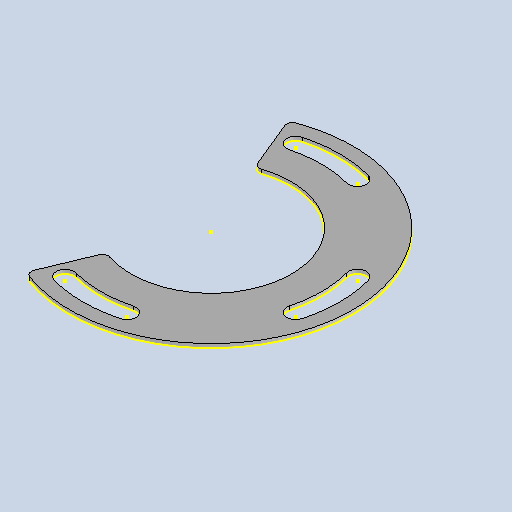
# Autodesk Inventor part: PNS 1707 funnel flange
Saved by Autodesk Inventor 2025.3 (Build 293356030, 356C)
## iProperties
Created: 2025-02-13
Part Number: PNS 1707 funnel flange
Material: Steel
Document SubType Name: Sheet Metal
Designer: admin
Mass: 720.962 g
Surface Area: 520.66 cm^2
Volume: 91.8424 cm^3
Density: 7.85 g/cm^3
Flat Pattern Width: 24.0684 cm
Flat Pattern Length: 28.4868 cm
Flat Pattern Area: 685.632 cm^2
Sheet Metal Rule: AISI304 4mm Die 32
Sheet Metal Width: 240,684 mm
Sheet Metal Length: 284,868 mm
Sheet Metal Area: 68563,227 mm^2
Appearance: Default
Author: pokla
Autodesk Inventor part; units mm, degrees
ref_plane "YZ Plane" through (0, 0, 0) normal (1, 0, 0) x (0, 1, 0)
ref_plane "XZ Plane" through (0, 0, 0) normal (0, 1, 0) x (-1, 0, 0)
ref_plane "XY Plane" through (0, 0, 0) normal (0, 0, 1) x (1, 0, 0)
sketch "Sketch2" plane through (0, 0, 0) normal (0, 0, 1) x (1, 0, 0)
  circle A0 centre (0, 0) radius 80.5
  circle A1 centre (0, 0) radius 142.5
  line L0 (0, 0) -> (-54.5324, 131.6528)
  line L1 (0, 0) -> (-54.5324, -131.6528)
  line L2 (0, 0) -> (-142.5, 0) construction
  point P0 (-30.806, -74.3723)
  point P1 (-30.806, 74.3723)
  dimension "d25" = 161
  dimension "d27" = 285
  dimension "d29" = 135
  measures "d25" diameter of A0
  measures "d27" diameter of A1
  measures "d29" angle of L1 L0
extrude "Plate2" add sketch "Sketch2" along normal blind 4 contours A0 L0 A1 L1 picked at (65.8732, 102.2302)
sketch "Sketch3" plane through (0, 0, 4) normal (0, 0, 1) x (1, 0, 0)
  circle A0 centre (0, 0) radius 120 construction
  arc A1 (31.0583, 115.9111) -> (-31.0583, 115.9111) centre (0, 0) ccw construction
  arc A2 (33.3877, 124.6044) -> (-33.3877, 124.6044) centre (0, 0) ccw
  arc A3 (28.7289, 107.2178) -> (-28.7289, 107.2178) centre (0, 0) ccw
  arc A4 (28.7289, 107.2178) -> (33.3877, 124.6044) centre (31.0583, 115.9111) ccw
  arc A5 (-33.3877, 124.6044) -> (-28.7289, 107.2178) centre (-31.0583, 115.9111) ccw
  line L0 (-31.0583, 115.9111) -> (0, 0)
  line L1 (0, 0) -> (31.0583, 115.9111)
  line L2 (0, 0) -> (0, 70.9879)
  dimension "d28" = 240
  dimension "d30" = 18
  dimension "d31" = 30
  constraints: 10 point on circle, 6 end point, 5 centre point, 4 tangent, 2 coincident, 1 vertical, 5 other
  measures "d30" diameter of A4
  measures "d31" angle of L1 L0
extrude "Cut1" cut sketch "Sketch3" against normal blind 4 contours A4 A3 A5 A2
pattern_circular "Circular Pattern1" count 4 over 360 about axis through (0, 0, 0) along (0, 0, 1) of "Cut1"
fillet "Corner Round1" radius 6 4 edges at (-54.5324, 131.6528, 2) (-30.806, 74.3723, 2) (-30.806, -74.3723, 2) (-54.5324, -131.6528, 2)
sketch "Sketch5" plane through (0, 0, 0) normal (0, 0, -1) x (-1, 0, 0)
  arc A0 (-107.2178, 28.7289) -> (-107.2178, -28.7289) centre (0, 0) ccw projected
  arc A1 (-124.6044, -33.3877) -> (-107.2178, -28.7289) centre (-115.9111, -31.0583) ccw projected
  arc A2 (-124.6044, 33.3877) -> (-124.6044, -33.3877) centre (0, 0) ccw projected
  arc A3 (-107.2178, 28.7289) -> (-124.6044, 33.3877) centre (-115.9111, 31.0583) ccw projected
  arc A4 (-28.7289, -107.2178) -> (28.7289, -107.2178) centre (0, 0) ccw projected
  arc A5 (33.3877, -124.6044) -> (28.7289, -107.2178) centre (31.0583, -115.9111) ccw projected
  arc A6 (-33.3877, -124.6044) -> (33.3877, -124.6044) centre (0, 0) ccw projected
  arc A7 (-28.7289, -107.2178) -> (-33.3877, -124.6044) centre (-31.0583, -115.9111) ccw projected
  arc A8 (28.7289, 107.2178) -> (-28.7289, 107.2178) centre (0, 0) ccw projected
  arc A9 (-33.3877, 124.6044) -> (-28.7289, 107.2178) centre (-31.0583, 115.9111) ccw projected
  arc A10 (33.3877, 124.6044) -> (-33.3877, 124.6044) centre (0, 0) ccw projected
  arc A11 (28.7289, 107.2178) -> (33.3877, 124.6044) centre (31.0583, 115.9111) ccw projected
  arc A12 (48.6927, -133.9226) -> (52.1858, -125.9877) centre (46.6425, -128.2838) ccw projected
  line L0 (33.0224, -79.7231) -> (52.1858, -125.9877) projected
  arc A13 (33.0224, -79.7231) -> (25.573, -76.33) centre (27.4791, -82.0192) ccw projected
  arc A14 (25.573, 76.33) -> (25.573, -76.33) centre (0, 0) ccw projected
  arc A15 (25.573, 76.33) -> (33.0224, 79.7231) centre (27.4791, 82.0192) ccw projected
  line L1 (52.1858, 125.9877) -> (33.0224, 79.7231) projected
  arc A16 (52.1858, 125.9877) -> (48.6927, 133.9226) centre (46.6425, 128.2838) ccw projected
  arc A17 (48.6927, 133.9226) -> (48.6927, -133.9226) centre (0, 0) ccw projected
  line L2 (14.6903, 87.3165) -> (-84.3637, 63.9504)
  line L3 (-84.3637, 63.9504) -> (-84.3637, -55.2862)
  line L4 (-84.3637, -55.2862) -> (17.3285, -91.5935)
  constraints: 6 end point, 1 vertical
equation "\"d17\" = Thickness"
equation "\"d14\" = Thickness"
equation "\"BendReliefWidth\" = Thickness"
equation "\"BendReliefDepth\" = 0.5 * Thickness"
equation "\"CornerReliefSize\" = 4 * Thickness"
equation "\"MinimumRemnant\" = 2 * Thickness"
equation "\"TransitionRadius\" = BendRadius"
equation "\"JacobiRadiusSize\" = BendRadius"
equation "\"GapSize\" = Thickness"
equation "\"Thickness\" = 4"
equation "\"BendRadius\" = 6"
body "Solid3"
